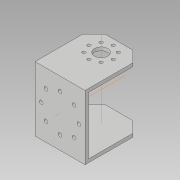
# Autodesk Inventor part: frame_mx108
Saved by Autodesk Inventor 2017 (Build 210142000, 142)
## iProperties
Part Number: frame_mx108
Material: Aluminium 6061
Document SubType Name: Modeling
Designer: Max
Density: 2.7 g/cm^3
Appearance: Vorgabe
Author: Max
Autodesk Inventor part; units mm, degrees
ref_plane "YZ Plane" through (0, 0, 0) normal (1, 0, 0) x (0, 1, 0)
ref_plane "XZ Plane" through (0, 0, 0) normal (0, 1, 0) x (-1, 0, 0)
ref_plane "XY Plane" through (0, 0, 0) normal (0, 0, 1) x (1, 0, 0)
sketch "Skizze1" plane through (0, 0, 0) normal (0, 1, 0) x (-1, 0, 0)
  line L0 (-22.5, 29) -> (22.5, 29)
  line L1 (22.5, 29) -> (22.5, -29)
  line L2 (22.5, -29) -> (-22.5, -29)
  line L3 (-22.5, -29) -> (-22.5, 29)
  line L4 (-22.5, 29) -> (22.5, -29) construction
  line L5 (22.5, 29) -> (-22.5, -29) construction
  point P0 (0, 0)
  dimension "d0" = 45
  dimension "d1" = 58
  constraints: 12 end point, 2 midpoint, 2 parallel, 1 horizontal, 1 perpendicular
  measures "d0" distance of L1.end L2.end
  measures "d1" distance of L0.end L1.end
extrude "Extrusion1" add sketch "Skizze1" along normal blind 3
sketch "Skizze2" plane through (0, 3, 0) normal (0, 1, 0) x (1, 0, 0)
  line L0 (-22.5, -29) -> (22.5, -29) projected
  line L1 (22.5, -29) -> (22.5, 29) projected
  line L2 (22.5, 29) -> (-22.5, 29) projected
  line L3 (-22.5, 29) -> (-22.5, -29) projected
  line L4 (-22.5, -29) -> (22.5, -29)
  line L5 (22.5, -29) -> (22.5, -26)
  line L6 (22.5, -26) -> (-22.5, -26)
  line L7 (-22.5, -26) -> (-22.5, -29)
  line L8 (22.5, 29) -> (-22.5, 29)
  line L9 (-22.5, 29) -> (-22.5, 26)
  line L10 (-22.5, 26) -> (22.5, 26)
  line L11 (22.5, 26) -> (22.5, 29)
  point P0 (0, 0)
  dimension "d4" = 3
  dimension "d5" = 3
  constraints: 16 end point, 4 parallel, 2 horizontal, 2 perpendicular, 2 point on line
  measures "d4" distance between parallel lines of L0 L6
  measures "d5" distance between parallel lines of L2 L10
extrude "Extrusion2" add sketch "Skizze2" along normal blind 50 contours L3 L6 L1 L0 | L3 L2 L1 L10
sketch "Skizze3" plane through (0, 3, 0) normal (0, 1, 0) x (1, 0, 0)
  line L0 (-22.5, -26) -> (22.5, -26) construction
  line L1 (22.5, -26) -> (22.5, 26) construction
  line L2 (22.5, 26) -> (-22.5, 26) construction
  line L3 (-22.5, 26) -> (-22.5, -26) construction
  line L4 (-22.5, -26) -> (22.5, 26) construction
  line L5 (-22.5, 26) -> (22.5, 26) construction
  line L6 (22.5, -26) -> (-22.5, 26) construction
  line L7 (16.9706, 0) -> (0, 16.9706) construction
  line L8 (0, 16.9706) -> (-16.9706, 0) construction
  line L9 (-16.9706, 0) -> (0, -16.9706) construction
  line L10 (0, -16.9706) -> (16.9706, 0) construction
  line L11 (16.9706, 0) -> (-16.9706, 0) construction
  line L12 (0, 16.9706) -> (0, -16.9706) construction
  circle A0 centre (0, 0) radius 18 construction
  line L13 (17.4913, 17.4913) -> (-17.5019, -17.5019) construction
  line L14 (16.4193, -16.4193) -> (-16.3603, 16.3603) construction
  point P0 (0, 0)
  point P1 (0, 0)
  point P2 (-12.7279, -12.7279)
  point P3 (12.7279, -12.7279)
  point P4 (12.7279, 12.7279)
  point P5 (-12.7279, 12.7279)
  dimension "d12" = 24
  dimension "d13" = 24
  dimension "d14" = 36
  constraints: 20 end point, 6 point on line, 5 midpoint, 4 point on circle, 3 perpendicular, 2 parallel, 1 centre point, 1 coincident, 1 horizontal
  measures "d12" distance of L8.end L9.end
  measures "d13" distance of L7.end L8.end
  measures "d14" diameter of A0
hole "Bohrung1" at (-16.9706, 3, 0) at (0, 3, -16.9706) at (16.9706, 3, 0) at (0, 3, 16.9706) at (-12.7279, 3, 12.7279) at (-12.7279, 3, -12.7279) at (12.7279, 3, -12.7279) at (12.7279, 3, 12.7279) direction (0, -1, 0) diameter 3.4 end through all clearance for "Inbusschraube ISO 4762" size "M3" standard "ISO"
sketch "Skizze4" plane through (-22.5, 0, 29) normal (0, 0, 1) x (1, 0, 0)
  line L0 (22.5, 0) -> (22.5, 74.8441) construction
  line L1 (0, 53) -> (45, 53) projected
  circle A0 centre (22.5, 37) radius 6
  line L2 (45, 0) -> (45, 52) projected
  line L3 (0, 52) -> (45, 52) projected
  line L4 (0, 0) -> (0, 52) projected
  point P0 (22.5, 48)
  dimension "d22" = 5
  dimension "d23" = 11
  dimension "d34" = 12
  constraints: 2 end point, 2 point on line, 1 centre point, 1 coincident, 1 vertical
  measures "d22" distance from line of L1 point (22.5, 48)
  measures "d23" distance of point (22.5, 48) point (22.5, 37)
  measures "d34" diameter of A0
hole "Bohrung2" at (0, 48, 29) direction (0, 0, -1) diameter 2.9 end up to face face through (-7.5, 19.6667, 26) facing (0, 0, -1) clearance for "Inbusschraube ISO 4762" size "M2.5" standard "ISO"
pattern_circular "Runde Anordnung1" count 8 over 360 about axis through (0, 37, 29) along (0, 0, 1) of "Bohrung2"
extrude "Extrusion3" cut sketch "Skizze4" against normal up to surface (3 mm away)
chamfer "Fase1" distance 10 angle 45 4 edges at (-22.5, 53, 27.5) (-22.5, 53, -27.5) (22.5, 53, 27.5) (22.5, 53, -27.5)
equation "\"d4\" = d5"
